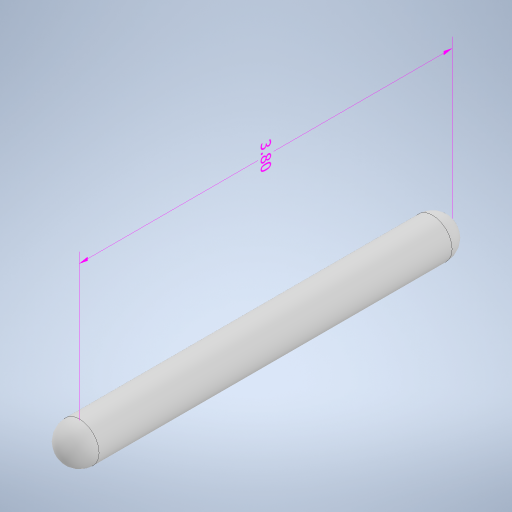
# Autodesk Inventor part: Single Wire
Saved by Autodesk Inventor 2023 (Build 270158000, 158)
## iProperties
Created: 2023-02-28
Part Number: Single Wire
Material: Generic
Document SubType Name: Modeling
Designer: 100KStarsun
Density: 1 g/cm^3
Appearance: Default
Author: 100KStarsun
Autodesk Inventor part; units mm, degrees
ref_plane "YZ Plane" through (0, 0, 0) normal (1, 0, 0) x (0, 1, 0)
ref_plane "XZ Plane" through (0, 0, 0) normal (0, 1, 0) x (-1, 0, 0)
ref_plane "XY Plane" through (0, 0, 0) normal (0, 0, 1) x (1, 0, 0)
sketch "Sketch4" plane through (0, 0, 0) normal (0, 1, 0) x (-1, 0, 0)
  line L0 (0, 0) -> (0, -101.6)
  line L1 (0, 0) -> (5.08, 0)
  line L2 (5.08, 0) -> (5.08, -101.6)
  line L3 (5.08, -101.6) -> (0, -101.6)
  line L4 (0, -101.6) -> (0, 0)
  dimension "d6" = 101.6
  dimension "d7" = 5.08
  constraints: 10 end point, 2 parallel, 1 horizontal, 1 perpendicular, 1 vertical
  measures "d6" distance of L0.start L0.end
  measures "d7" distance of L2.end L3.end
revolve "Revolution1" add sketch "Sketch4" angle 360 about axis through (0, 0, 0) along (0, 0, -1)
fillet "Fillet1" radius 5.08 1 edges at (5.08, 0, 0)
fillet "Fillet2" radius 5.08 1 edges at (5.08, 0, -101.6)
